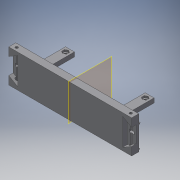
# Autodesk Inventor part: Case_bottom_back
Saved by Autodesk Inventor 2016 SP2 (Build 200236200, 236)
## iProperties
Created: 2018-06-26
Part Number: Case_bottom_back
Material: Generisch
Document SubType Name: Modeling
Designer: Nils
Density: 1 g/cm^3
Appearance: Vorgabe
Author: Nils
Autodesk Inventor part; units mm, degrees
ref_plane "YZ Plane" through (0, 0, 0) normal (1, 0, 0) x (0, 1, 0)
ref_plane "XZ Plane" through (0, 0, 0) normal (0, 1, 0) x (-1, 0, 0)
ref_plane "XY Plane" through (0, 0, 0) normal (0, 0, 1) x (1, 0, 0)
sketch "Skizze1" plane through (0, 0, 0) normal (1, 0, 0) x (0, 1, 0)
  line L0 (164.688, -161.6072) -> (164.688, -152.3072) projected
  line L1 (156.688, -152.3072) -> (156.688, -161.7307) projected
  line L2 (156.688, -152.3072) -> (164.688, -152.3072) projected
  line L3 (164.688, -161.6072) -> (166.188, -161.6072) projected
  line L4 (166.188, -161.6072) -> (166.188, -162.1072) projected
  line L5 (166.188, -162.1072) -> (165.438, -162.8572) projected
  line L6 (156.688, -180.1837) -> (156.688, -189.6072) projected
  line L7 (164.688, -189.6072) -> (156.688, -189.6072) projected
  line L8 (164.688, -189.6072) -> (164.688, -187.6072)
  line L9 (164.688, -187.6072) -> (165.688, -187.6072)
  line L10 (165.688, -187.6072) -> (165.688, -186.6072)
  line L11 (165.688, -186.6072) -> (164.688, -186.6072)
  line L12 (156.688, -180.1837) -> (156.688, -161.7307)
  line L13 (164.688, -186.6072) -> (164.688, -163.6072)
  line L14 (164.688, -163.6072) -> (165.438, -162.8572)
  point P0 (0, 0)
  dimension "d19" = 2
  dimension "d20" = 1
  dimension "d21" = 1
  constraints: 14 end point, 3 perpendicular, 3 vertical, 1 collinear, 1 point on line
  measures "d19" distance of L7.start L8.end
  measures "d20" distance of L8.end L9.end
  measures "d21" distance of L9.end L10.end
extrude "Extrusion1" add sketch "Skizze1" along normal blind 69.4
sketch "Skizze2" plane through (0, 156.688, -189.6072) normal (0, -1, 0) x (1, 0, 0)
  line L0 (0, 27.8765) -> (10, 33.65)
  line L1 (10, 33.65) -> (10, 3.65)
  line L2 (10, 3.65) -> (0, 9.4235)
  line L3 (0, 0) -> (0, 26.75) projected
  line L4 (0, 27.8765) -> (0, 9.4235)
  line L5 (-0.1, 9.3658) -> (10.1, 3.4768)
  line L6 (10.1, 3.4768) -> (10.1, 33.8232)
  line L7 (10.1, 33.8232) -> (-0.1, 27.9342)
  line L8 (-0.1, 27.9342) -> (-0.1, 9.3658)
  line L9 (10, 33.65) -> (0, 27.8765) projected
  line L10 (10, 33.65) -> (0, 27.8765) projected
  line L11 (10, 3.65) -> (6.118, 5.8913) projected
  line L12 (0, 9.4235) -> (10, 3.65) projected
  point P0 (0, 189.6072)
  point P1 (-212.8594, 35.25)
  point P2 (-212.8594, 5.25)
  point P3 (-222.8594, 29.4765)
  point P4 (-222.8594, 11.0235)
  dimension "d7" = 0.1
  constraints: 16 end point, 3 collinear, 1 equal length, 1 point on line, 1 vertical, 8 other
  measures "d7" distance between parallel lines of L6 L1
extrude "Extrusion2" cut sketch "Skizze2" against normal blind 5 contours L0 L1 L2 L3 L4 | L8 L7 L6 L5
sketch "Skizze3" plane through (0, 156.688, -152.3072) normal (0, 0, 1) x (1, 0, 0)
  circle A0 centre (5, 4) radius 1.5 projected
  point P0 (0, -156.688)
extrude "Extrusion3" cut sketch "Skizze3" against normal blind 35
sketch "Skizze11" plane through (0, 164.688, -163.6072) normal (0, 1, 0) x (1, 0, 0)
  line L0 (2.15, 8.75) -> (7.85, 8.75) projected
  line L1 (2.15, 5.95) -> (2.15, 8.75) projected
  line L2 (7.85, 8.75) -> (7.85, 5.95) projected
  line L3 (7.85, 5.95) -> (2.15, 5.95) projected
  point P0 (0, -163.6072)
extrude "Extrusion12" cut sketch "Skizze11" against normal blind 4.45
sketch "Skizze12" plane through (0, 164.688, -163.6072) normal (0, 1, 0) x (1, 0, 0)
  line L0 (29.0604, 1.25) -> (19.4, 1.25) construction
  line L1 (19.4, 14.2294) -> (19.4, -8.7706) construction
  line L2 (12.6604, 1.25) -> (34.3604, 1.25) construction
  line L3 (0, 0) -> (69.4, 0) projected
  line L4 (0, 23) -> (0, 0) projected
  line L5 (0, -11.3) -> (69.4, -11.3) projected
  line L6 (19.4, 1.25) -> (29.4, 1.25)
  line L7 (29.4, 1.25) -> (29.4, 6.25)
  line L8 (29.4, 6.25) -> (19.4, 6.25)
  line L9 (19.4, 6.25) -> (19.4, 1.25)
  point P0 (0, -163.6072)
  dimension "d53" = 19.4
  dimension "d54" = 12.55
  dimension "d55" = 10
  dimension "d56" = 5
  constraints: 14 end point, 3 point on line, 2 parallel, 1 horizontal, 1 perpendicular
  measures "d53" distance between parallel lines of L1 L4
  measures "d54" distance between parallel lines of L5 L0
  measures "d55" distance of L8.end L7.end
  measures "d56" distance of L7.end L6.end
extrude "Extrusion13" add sketch "Skizze12" along normal blind 36.75
sketch "Skizze13" plane through (19.4, 164.688, -164.8572) normal (0, 0, 1) x (1, 0, 0)
  circle A0 centre (5, 31.75) radius 1.55
  line L0 (0, 0) -> (0, 36.75) projected
  line L1 (0, 36.75) -> (10, 36.75) projected
  dimension "d59" = 3.1
  dimension "d60" = 5
  dimension "d61" = 5
  constraints: 1 centre point
  measures "d59" diameter of A0
  measures "d60" distance from line of A0.centre L0
  measures "d61" distance from line of A0.centre L1
extrude "Extrusion14" cut sketch "Skizze13" against normal blind 5
sketch "Skizze14" plane through (19.4, 164.688, -164.8572) normal (0, 0, 1) x (1, 0, 0)
  circle A0 centre (5, 31.75) radius 1.55 construction
  line L0 (5, 28.4591) -> (2.15, 30.1046)
  line L1 (2.15, 30.1046) -> (2.15, 33.3954)
  line L2 (2.15, 33.3954) -> (5, 35.0409)
  line L3 (5, 35.0409) -> (7.85, 33.3954)
  line L4 (7.85, 33.3954) -> (7.85, 30.1046)
  line L5 (7.85, 30.1046) -> (5, 28.4591)
  point P0 (-19.4, -164.688)
  dimension "d64" = 5.7
  constraints: 12 end point, 1 coincident, 1 vertical, 13 other
  measures "d64" distance between parallel lines of L1 L4
extrude "Extrusion15" cut sketch "Skizze14" against normal blind 2.2
mirror "Spiegeln3" about plane through (69.4, 160.9198, -171.097) normal (1, 0, 0) of "Extrusion15", "Extrusion14", "Extrusion13", "Extrusion12", "Extrusion3", "Extrusion2", "Extrusion1"
ref_plane "Arbeitsebene1" through (69.4, 156.688, -152.3072) normal (1, 0, 0) x (0, 0, -1)
sketch "Skizze15" plane through (0, 0, 0) normal (0, 0, 1) x (1, 0, 0)
  point P0 (0, 0)
equation "\"d61\" = d60"
